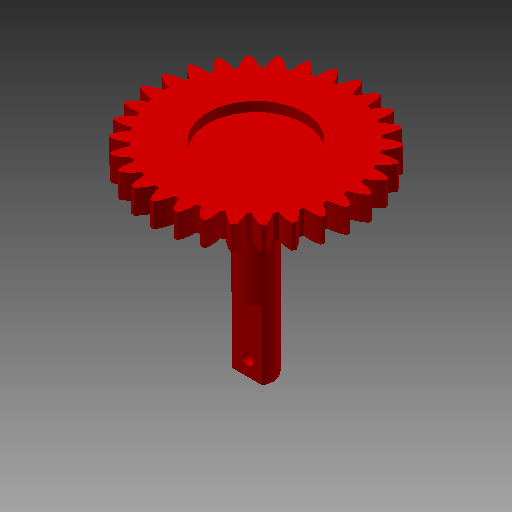
# Autodesk Inventor part: Front Gear
Saved by Autodesk Inventor 2018 (Build 220112000, 112)
## iProperties
Created: 2014-09-16
Part Number: Front Gear
Material: Generic
Document SubType Name: Modeling
Designer: loust
Density: 1 g/cm^3
Appearance: Default(1)
Author: loust
Autodesk Inventor part; units mm, degrees
ref_plane "YZ Plane" through (0, 0, 0) normal (1, 0, 0) x (0, 1, 0)
ref_plane "XZ Plane" through (0, 0, 0) normal (0, 1, 0) x (-1, 0, 0)
ref_plane "XY Plane" through (0, 0, 0) normal (0, 0, 1) x (1, 0, 0)
sketch "Sketch1" plane through (0, 0, 0) normal (0, 1, 0) x (-1, 0, 0)
  circle A0 centre (0, 0) radius 18.5
  dimension "d0" = 37
  constraints: 1 centre point, 1 coincident
  measures "d0" diameter of A0
extrude "Extrusion1" add sketch "Sketch1" along normal blind 5
sketch "Sketch2" plane through (0, 5, 0) normal (0, 1, 0) x (1, 0, 0)
  circle A0 centre (0, 0) radius 18.5 projected
  line L0 (-0.35, 21.5) -> (0.35, 21.5)
  line L1 (0, 29.5757) -> (0, -26.5304) projected
  arc A1 (-0.35, 21.5) -> (-1.5, 18.4391) centre (6.2621, 17.2693) ccw
  arc A2 (1.5, 18.4391) -> (0.35, 21.5) centre (-6.2623, 17.2692) ccw
  arc A3 (1.5, 18.4391) -> (0, -18.5) centre (0, 0) ccw
  point P0 (0, 18.5)
  dimension "d4" = 0.7
  dimension "d5" = 0.35
  dimension "d6" = 3
  dimension "d7" = 7.8498
  dimension "d8" = 7.85
  constraints: 9 point on circle, 3 centre point, 2 end point, 2 point on line, 1 coincident, 1 concentric, 1 horizontal
  measures "d4" distance of L0.start L0.end
  measures "d5" distance from line of L1 L0.end
  measures "d6" distance edge to line of A0 L0
  measures "d7" radius of A1
  measures "d8" radius of A2
extrude "Extrusion2" add sketch "Sketch2" against normal up to surface (5 mm away) contours A0 L1 L0 A2 | A0 A1 L0 L1
pattern_circular "Circular Pattern1" count 30 over 360 about axis through (0, -10, 0) along (0, 1, 0) of "Extrusion2"
sketch "Sketch4" plane through (0, 5, 0) normal (0, 1, 0) x (1, 0, 0)
  arc A0 (2.3665, 18.348) -> (1.5, 18.4391) centre (0, 0) ccw projected
  circle A1 centre (0, 0) radius 10
  dimension "d14" = 20
  constraints: 1 centre point, 1 coincident
  measures "d14" diameter of A1
extrude "Extrusion3" cut sketch "Sketch4" against normal blind 2
sketch "Sketch5" plane through (0, 0, 0) normal (0, -1, 0) x (1, 0, 0)
  arc A0 (-2.3665, -18.348) -> (-1.5, -18.4391) centre (0, 0) ccw projected
  circle A1 centre (0, 0) radius 3.6
  dimension "d17" = 7.2
  constraints: 1 centre point, 1 coincident
  measures "d17" diameter of A1
extrude "Extrusion4" add sketch "Sketch5" along normal blind 36.4
sketch "Sketch6" plane through (0, -36.4, 0) normal (0, -1, 0) x (1, 0, 0)
  circle A0 centre (0, 0) radius 3.6 projected
  line L0 (3.1177, 1.8) -> (-3.1177, 1.8)
  arc A1 (3.1177, 1.8) -> (-3.1177, 1.8) centre (0, 0) ccw
  dimension "d20" = 1.8
  constraints: 4 point on circle, 2 end point, 1 centre point, 1 coincident, 1 concentric, 1 horizontal
  measures "d20" distance from line of A0.centre L0
extrude "Extrusion5" cut sketch "Sketch6" against normal blind 14.4 contours L0 A0 picked at (-0.8728, 2.0235)
sketch "Sketch7" plane through (-3.1177, -36.4, 1.8) normal (0, 0, 1) x (1, 0, 0)
  line L0 (6.2354, 0) -> (0, 0) projected
  circle A0 centre (3.1177, 3.2) radius 1.2
  point P0 (3.1177, 36.4)
  dimension "d23" = 2.4
  dimension "d24" = 3.2
  constraints: 1 centre point
  measures "d23" diameter of A0
  measures "d24" distance from line of L0 A0.centre
extrude "Extrusion6" cut sketch "Sketch7" against normal through all
body "Solid1"
